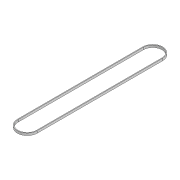
# Autodesk Inventor part: Belt
Saved by Autodesk Inventor 2020 (Build 240168000, 168)
## iProperties
Created: 2020-11-06
Part Number: Belt
Material: Generic
Document SubType Name: Modeling
Designer: ferrerx
Density: 1 g/cm^3
Appearance: Default
Author: ferrerx
Autodesk Inventor part; units mm, degrees
ref_plane "YZ Plane" through (0, 0, 0) normal (1, 0, 0) x (0, 1, 0)
ref_plane "XZ Plane" through (0, 0, 0) normal (0, 1, 0) x (-1, 0, 0)
ref_plane "XY Plane" through (0, 0, 0) normal (0, 0, 1) x (1, 0, 0)
sketch "Sketch1" plane through (0, 0, 0) normal (0, 1, 0) x (-1, 0, 0)
  arc A0 (25.21, 0) -> (-25.21, 0) centre (0, 0) ccw
  arc A1 (27.21, 0) -> (-27.21, 0) centre (0, 0) ccw
  arc A2 (-25.21, -343) -> (25.21, -343) centre (0, -343) ccw
  arc A3 (-27.21, -343) -> (27.21, -343) centre (0, -343) ccw
  line L0 (0, 0) -> (0, -343) construction
  line L1 (27.21, 0) -> (27.21, -343)
  line L2 (-27.21, 0) -> (-27.21, -343)
  line L3 (25.21, 0) -> (25.21, -343)
  line L4 (-25.21, 0) -> (-25.21, -343)
  dimension "d0" = 343
  dimension "d1" = 50.42
  dimension "d2" = 50.42
  dimension "d3" = 2
  dimension "d4" = 2
  constraints: 10 end point, 8 point on circle, 4 centre point, 4 tangent, 3 coincident, 1 vertical
  measures "d0" distance of L0.start L0.end
  measures "d1" diameter of A0
  measures "d2" diameter of A2
  measures "d3" radial gap between concentric circles of A1 A0
  measures "d4" radial gap between concentric circles of A3 A2
extrude "Extrusion1" add sketch "Sketch1" along normal blind 6
body "Solid1"
